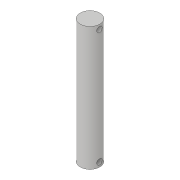
# Autodesk Inventor part: SUS-ShockAbsorber
Saved by Autodesk Inventor 2019.4 (Build 234330000, 330)
## iProperties
Created: 2020-02-15
Part Number: SUS-ShockAbsorber
Material: Generic
Document SubType Name: Modeling
Designer: Lord of Xy
Density: 1 g/cm^3
Appearance: Default
Author: Lord of Xy
Autodesk Inventor part; units mm, degrees
ref_plane "YZ Plane" through (0, 0, 0) normal (1, 0, 0) x (0, 1, 0)
ref_plane "XZ Plane" through (0, 0, 0) normal (0, 1, 0) x (-1, 0, 0)
ref_plane "XY Plane" through (0, 0, 0) normal (0, 0, 1) x (1, 0, 0)
sketch "Sketch1" plane through (0, 0, 0) normal (0, 1, 0) x (-1, 0, 0)
  circle A0 centre (0, 0) radius 8.5
  dimension "d0" = 17
  constraints: 1 centre point, 1 coincident
  measures "d0" diameter of A0
extrude "Extrusion1" add sketch "Sketch1" along normal mid plane 108
sketch "Sketch2" plane through (0, 0, 0) normal (1, 0, 0) x (0, 1, 0)
  line L0 (50, 0) -> (-50, 0)
  point P0 (0, 0)
  point P1 (0, 0)
  dimension "d3" = 100
  constraints: 2 end point, 1 coincident, 1 horizontal, 1 midpoint
  measures "d3" distance of L0.start L0.end
hole "Hole1" at (0, 50, 0) at (0, -50, 0) direction (1, 0, 0) diameter 4.7625 end through all both
body "Solid1"
